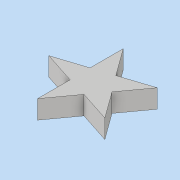
# Autodesk Inventor part: Деталь3
Saved by Autodesk Inventor 2019 (Build 230136000, 136)
## iProperties
Created: 2021-02-22
Part Number: Деталь3
Material: Типовые
Document SubType Name: Modeling
Designer: Kurbatova
Density: 1 g/cm^3
Appearance: По умолчанию
Author: Kurbatova
Autodesk Inventor part; units mm, degrees
ref_plane "YZ Plane" through (0, 0, 0) normal (1, 0, 0) x (0, 1, 0)
ref_plane "XZ Plane" through (0, 0, 0) normal (0, 1, 0) x (-1, 0, 0)
ref_plane "XY Plane" through (0, 0, 0) normal (0, 0, 1) x (1, 0, 0)
sketch "Эскиз1" plane through (0, 0, 0) normal (0, 1, 0) x (-1, 0, 0)
  circle A0 centre (141.9995, 431.0309) radius 94.7983
  line L0 (141.9995, 613.3951) -> (141.9995, 248.6146)
  line L1 (141.9995, 431.0309) -> (232.158, 401.7366)
  line L2 (170.6201, 521.4056) -> (170.6201, 453.1496)
  line L3 (171.4591, 340.9262) -> (171.4591, 410.4158)
  line L4 (171.4591, 340.9262) -> (130.4621, 397.3537)
  line L5 (64.7967, 486.044) -> (129.6246, 464.9802)
  line L6 (64.7967, 486.044) -> (104.7661, 431.0309)
  line L7 (170.6201, 453.1496) -> (236.7967, 431.4888)
  line L8 (236.7967, 431.4888) -> (171.4591, 410.4158)
  line L9 (130.4621, 397.3537) -> (64.7967, 376.0177)
  line L10 (64.7967, 376.0177) -> (104.7661, 431.0309)
  line L11 (170.6201, 521.4056) -> (129.6246, 464.9802)
  point P0 (141.9995, 431.0049)
  dimension "d22" = 172
  dimension "d24" = 172
  dimension "d27" = 72
  dimension "d41" = 36
  dimension "d43" = 36
  dimension "d44" = 36
  dimension "d45" = 36
  dimension "d46" = 36
  constraints: 24 end point, 6 point on circle, 3 vertical, 1 centre point, 1 midpoint, 1 parallel, 1 point on line
  measures "d22" horizontal distance of L7.end L9.end
  measures "d24" horizontal distance of L7.end L5.start
  measures "d27" angle of L0 L1
  measures "d41" angle of L4 L3
  measures "d43" angle of L11 L2
  measures "d44" angle of L10 L9
  measures "d45" angle of L5 L6
  measures "d46" angle of L7 L8
extrude "Выдавливание1" add sketch "Эскиз1" against normal blind 39 contours L8 L1 L0 L11 L2 L7 | L8 L3 L4 L0 L1 | L0 L4 L9 L10 L6 L5 L11
